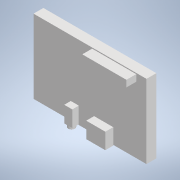
# Autodesk Inventor part: RaspberryPi3_Screen
Saved by Autodesk Inventor 2021 (Build 250183000, 183)
## iProperties
Created: 2021-04-21
Part Number: RaspberryPi3_Screen
Material: Generic
Document SubType Name: Modeling
Designer: trent
Density: 1 g/cm^3
Appearance: Default
Author: trent
Autodesk Inventor part; units mm, degrees
ref_plane "YZ Plane" through (0, 0, 0) normal (1, 0, 0) x (0, 1, 0)
ref_plane "XZ Plane" through (0, 0, 0) normal (0, 1, 0) x (-1, 0, 0)
ref_plane "XY Plane" through (0, 0, 0) normal (0, 0, 1) x (1, 0, 0)
sketch "Sketch1" plane through (0, 0, 0) normal (0, 0, 1) x (1, 0, 0)
  line L0 (0, 0) -> (85.75, 0)
  line L1 (85.75, 0) -> (85.75, 56)
  line L2 (85.75, 56) -> (0, 56)
  line L3 (0, 56) -> (0, 0)
  dimension "d0" = 85.75
  dimension "d1" = 56
  constraints: 8 end point, 2 parallel, 1 horizontal, 1 perpendicular
  measures "d0" distance of L1.end L2.end
  measures "d1" distance of L0.end L1.end
extrude "Extrusion1" add sketch "Sketch1" along normal blind 7.5
sketch "Sketch3" plane through (0, 0, 7.5) normal (0, 0, 1) x (1, 0, 0)
  line L0 (78, 55.25) -> (44.5, 55.25)
  line L1 (44.5, 55.25) -> (44.5, 50.25)
  line L2 (44.5, 50.25) -> (78, 50.25)
  line L3 (78, 50.25) -> (78, 55.25)
  line L4 (85.75, 56) -> (0, 56) projected
  line L5 (85.75, 0) -> (85.75, 56) projected
  point P0 (0, 0)
  dimension "d19" = 33.5
  dimension "d20" = 5
  dimension "d21" = 0.75
  dimension "d22" = 7.75
  constraints: 8 end point, 2 parallel, 1 horizontal, 1 perpendicular
  measures "d19" distance of L0.start L0.end
  measures "d20" distance of L0.end L1.end
  measures "d21" distance between parallel lines of L4 L0
  measures "d22" distance between parallel lines of L5 L3
extrude "Extrusion3" add sketch "Sketch3" along normal blind 7.5
sketch "Sketch4" plane through (0, 0, 7.5) normal (0, 0, 1) x (1, 0, 0)
  line L0 (46, 11.65) -> (60.5, 11.65)
  line L1 (60.5, 11.65) -> (60.5, -0.5)
  line L2 (60.5, -0.5) -> (46, -0.5)
  line L3 (46, -0.5) -> (46, 11.65)
  line L4 (0, 0) -> (85.75, 0) projected
  line L5 (85.75, 0) -> (85.75, 56) projected
  dimension "d25" = 14.5
  dimension "d26" = 12.15
  dimension "d28" = 0.5
  dimension "d29" = 25.25
  constraints: 8 end point, 2 parallel, 1 horizontal, 1 perpendicular
  measures "d25" distance of L1.end L2.end
  measures "d26" distance of L0.end L1.end
  measures "d28" distance between parallel lines of L2 L4
  measures "d29" distance between parallel lines of L5 L1
extrude "Extrusion4" add sketch "Sketch4" along normal blind 6
sketch "Sketch5" plane through (0, 0, 7.5) normal (0, 0, 1) x (1, 0, 0)
  line L0 (28.3, 12.75) -> (34.4, 12.75)
  line L1 (34.4, 12.75) -> (34.4, 0.5)
  line L2 (34.4, 0.5) -> (28.3, 0.5)
  line L3 (28.3, 0.5) -> (28.3, 12.75)
  line L4 (0, 0) -> (46, 0) projected
  line L5 (0, 56) -> (0, 0) projected
  dimension "d32" = 12.25
  dimension "d33" = 6.1
  dimension "d35" = 28.3
  dimension "d36" = 0.5
  constraints: 8 end point, 2 parallel, 1 horizontal, 1 perpendicular
  measures "d32" distance of L2.end L0.start
  measures "d33" distance of L0.start L0.end
  measures "d35" distance between parallel lines of L5 L3
  measures "d36" distance between parallel lines of L4 L2
extrude "Extrusion5" add sketch "Sketch5" along normal blind 5
sketch "Sketch6" plane through (28.3, 0.5, 7.5) normal (0, -1, 0) x (1, 0, 0)
  line L0 (6.1, 5) -> (0, 5) projected
  line L1 (3.05, 5) -> (3.05, 2.5)
  circle A0 centre (3.05, 2.5) radius 2.5
  point P0 (-28.3, -7.5)
  dimension "d39" = 2.5
  dimension "d40" = 5
  constraints: 2 end point, 1 centre point, 1 coincident, 1 midpoint, 1 vertical
  measures "d39" distance of L1.start L1.end
  measures "d40" diameter of A0
extrude "Extrusion6" add sketch "Sketch6" along normal blind 2
body "Solid1"
